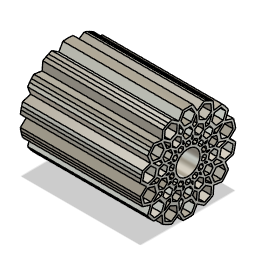
chevron + honeycomb v2 (Autodesk Fusion 360 archive; units mm, degrees)
design "honeycomb support"
Autodesk Fusion 360 part; units mm, degrees
sketch "Sketch1" plane through (0, 0, 0) normal (1, 0, 0) x (0, 0, -1)
  circle A0 centre (0, 0) radius 5
  circle A1 centre (0, 0) radius 20
  line L0 (0, 20.0404) -> (0, 18.9404) construction
  line L1 (0, 0) -> (0, 38.9808) construction
  line L2 (0, 13.1782) -> (0, 12.6782) construction
  line L3 (0, 8.1981) -> (0, 7.9981) construction
  line L4 (0, 5) -> (0, 5.5) construction
  line L5 (0, 8.0981) -> (0, 8.5981) construction
  line L6 (0, 12.9282) -> (0, 13.3) construction
  line L7 (0, 12.9282) -> (0, 13.4282) construction
  circle A2 centre (0, 0) radius 6
  line L8 (3.5471, 15.5409) -> (2.0387, 12.9282)
  line L9 (-2.0387, 12.9282) -> (-3.5471, 15.5409)
  line L10 (-3.8476, 16.8573) -> (-2.0968, 19.8898)
  line L11 (2.0968, 19.8898) -> (3.8476, 16.8573)
  line L12 (-2.6325, 11.5337) -> (-1.933, 12.7452)
  line L13 (1.933, 12.7452) -> (2.6325, 11.5337)
  line L14 (-1.7007, 7.4514) -> (-1.433, 7.9151)
  line L15 (1.433, 7.9151) -> (1.7007, 7.4514)
  line L16 (1.4613, 13.9282) -> (-1.4613, 13.9282)
  line L17 (-1.4613, 13.9282) -> (-2.9226, 16.4593)
  line L18 (-2.9226, 16.4593) -> (-1.4613, 18.9904)
  line L19 (-1.4613, 18.9904) -> (1.4613, 18.9904)
  line L20 (1.4613, 18.9904) -> (2.9226, 16.4593)
  line L21 (2.9226, 16.4593) -> (1.4613, 13.9282)
  line L22 (1.0191, 8.9981) -> (-1.0191, 8.9981)
  line L23 (-1.0191, 8.9981) -> (-2.0381, 10.7631)
  line L24 (-2.0381, 10.7631) -> (-1.0191, 12.5282)
  line L25 (-1.0191, 12.5282) -> (1.0191, 12.5282)
  line L26 (1.0191, 12.5282) -> (2.0381, 10.7631)
  line L27 (2.0381, 10.7631) -> (1.0191, 8.9981)
  line L28 (-0.6706, 5.9624) -> (-1.1536, 6.799)
  line L29 (-1.1536, 6.799) -> (-0.5768, 7.7981)
  line L30 (-0.5768, 7.7981) -> (0.5768, 7.7981)
  line L31 (0.5768, 7.7981) -> (1.1536, 6.799)
  line L32 (1.1536, 6.799) -> (0.6706, 5.9624)
  line L33 (1.5387, 8.0981) -> (1.4302, 7.9102)
  line L34 (1.5387, 8.0981) -> (1.7557, 8.0981) construction
  line L35 (-1.5387, 8.0981) -> (-1.433, 7.9151)
  line L36 (-1.5387, 8.0981) -> (-1.3274, 8.0981) construction
  line L37 (-2.0387, 12.9282) -> (-1.9268, 12.7345)
  line L38 (-2.0387, 12.9282) -> (-1.815, 12.9282) construction
  line L39 (2.0387, 12.9282) -> (1.933, 12.7452)
  line L40 (-7.4461, 10.7634) -> (-7.2613, 10.6374)
  line L41 (-7.4461, 10.7634) -> (-9.9388, 12.4628)
  line L42 (-10.7806, 13.5185) -> (-10.5103, 17.1262)
  line L43 (-10.5103, 17.1262) -> (-6.8367, 18.8953)
  line L44 (-6.8367, 18.8953) -> (-3.8476, 16.8573)
  line L45 (-3.7726, 12.5325) -> (-3.7883, 12.3217)
  line L46 (-3.7883, 12.3217) -> (-2.6325, 11.5337)
  line L47 (-2.1273, 7.9637) -> (-2.1435, 7.7473)
  line L48 (-3.5471, 15.5409) -> (-3.7726, 12.5325)
  line L49 (-2.1431, 7.753) -> (-1.7007, 7.4514)
  line L50 (-4.7653, 5.9755) -> (-4.7253, 6.5095)
  line L51 (-4.8999, 6.6285) -> (-4.7253, 6.5095)
  line L52 (-7.3761, 9.2493) -> (-7.2715, 10.6443)
  line L53 (-4.5176, 11.7297) -> (-2.8337, 10.5816)
  line L54 (-2.8337, 10.5816) -> (-2.986, 8.5491)
  line L55 (-2.986, 8.5491) -> (-4.8223, 7.6648)
  line L56 (-4.8223, 7.6648) -> (-6.5062, 8.8129)
  line L57 (-6.3539, 10.8454) -> (-4.5176, 11.7297)
  line L58 (-6.5062, 8.8129) -> (-6.3539, 10.8454)
  line L59 (-9.5562, 16.4757) -> (-6.923, 17.7438)
  line L60 (-6.923, 17.7438) -> (-4.5082, 16.0974)
  line L61 (-4.5082, 16.0974) -> (-4.7266, 13.1829)
  line L62 (-4.7266, 13.1829) -> (-7.3598, 11.9148)
  line L63 (-9.7746, 13.5612) -> (-9.5562, 16.4757)
  line L64 (-7.3598, 11.9148) -> (-9.7746, 13.5612)
  line L65 (-2.8638, 7.2761) -> (-1.9106, 6.6262)
  line L66 (-1.9106, 6.6262) -> (-1.9828, 5.6629)
  line L67 (-3.1911, 5.081) -> (-3.9893, 5.6252)
  line L68 (-3.9031, 6.7756) -> (-2.8638, 7.2761)
  line L69 (-3.9893, 5.6252) -> (-3.9031, 6.7756)
  line L70 (-11.3788, 6.4667) -> (-11.1576, 6.4334)
  line L71 (-11.3788, 6.4667) -> (-14.3619, 6.9163)
  line L72 (-15.5785, 7.5022) -> (-16.9002, 10.8699)
  line L73 (-16.9002, 10.8699) -> (-14.358, 14.0577)
  line L74 (-14.358, 14.0577) -> (-10.7806, 13.5185)
  line L75 (-8.8366, 9.6545) -> (-8.7594, 9.4578)
  line L76 (-8.7594, 9.4578) -> (-7.3761, 9.2493)
  line L77 (-5.372, 6.2521) -> (-5.2927, 6.0501)
  line L78 (-9.9388, 12.4628) -> (-8.8366, 9.6545)
  line L79 (-5.2948, 6.0553) -> (-4.7653, 5.9755)
  line L80 (-6.8861, 3.3162) -> (-7.0817, 3.8146)
  line L81 (-7.2907, 3.8461) -> (-7.0817, 3.8146)
  line L82 (-10.6587, 5.133) -> (-11.1698, 6.4352)
  line L83 (-9.1596, 8.6079) -> (-7.1442, 8.3042)
  line L84 (-7.1442, 8.3042) -> (-6.3996, 6.4069)
  line L85 (-6.3996, 6.4069) -> (-7.6704, 4.8135)
  line L86 (-7.6704, 4.8135) -> (-9.6857, 5.1172)
  line L87 (-10.4303, 7.0145) -> (-9.1596, 8.6079)
  line L88 (-9.6857, 5.1172) -> (-10.4303, 7.0145)
  line L89 (-15.7584, 10.6978) -> (-13.9362, 12.9828)
  line L90 (-13.9362, 12.9828) -> (-11.0462, 12.5472)
  line L91 (-11.0462, 12.5472) -> (-9.9784, 9.8266)
  line L92 (-9.9784, 9.8266) -> (-11.8006, 7.5416)
  line L93 (-14.6906, 7.9772) -> (-15.7584, 10.6978)
  line L94 (-11.8006, 7.5416) -> (-14.6906, 7.9772)
  line L95 (-5.7372, 5.313) -> (-4.5965, 5.141)
  line L96 (-4.5965, 5.141) -> (-4.2435, 4.2418)
  line L97 (-5.0797, 3.1932) -> (-6.035, 3.3372)
  line L98 (-6.4564, 4.4111) -> (-5.7372, 5.313)
  line L99 (-6.035, 3.3372) -> (-6.4564, 4.4111)
  line L100 (-13.0577, 0.8892) -> (-12.844, 0.9552)
  line L101 (-13.0577, 0.8892) -> (-15.9405, 0)
  line L102 (-17.2908, 0) -> (-19.9428, 2.4607)
  line L103 (-19.9428, 2.4607) -> (-19.0355, 6.4358)
  line L104 (-19.0355, 6.4358) -> (-15.5785, 7.5022)
  line L105 (-12.1504, 4.8644) -> (-11.9955, 4.7206)
  line L106 (-11.9955, 4.7206) -> (-10.6587, 5.133)
  line L107 (-7.5527, 3.3021) -> (-7.3936, 3.1545)
  line L108 (-14.3619, 6.9163) -> (-12.1504, 4.8644)
  line L109 (-7.3977, 3.1584) -> (-6.8861, 3.3162)
  line L110 (-7.643, 0) -> (-8.0355, 0.3642)
  line L111 (-8.2374, 0.3019) -> (-8.0355, 0.3642)
  line L112 (-11.8303, 0) -> (-12.8558, 0.9515)
  line L113 (-11.9873, 3.7813) -> (-10.0398, 4.382)
  line L114 (-10.0398, 4.382) -> (-8.5457, 2.9958)
  line L115 (-8.5457, 2.9958) -> (-8.9992, 1.0088)
  line L116 (-8.9992, 1.0088) -> (-10.9468, 0.408)
  line L117 (-12.4409, 1.7943) -> (-11.9873, 3.7813)
  line L118 (-10.9468, 0.408) -> (-12.4409, 1.7943)
  line L119 (-18.8394, 2.8011) -> (-18.1891, 5.6504)
  line L120 (-18.1891, 5.6504) -> (-15.3963, 6.5119)
  line L121 (-15.3963, 6.5119) -> (-13.2538, 4.524)
  line L122 (-13.2538, 4.524) -> (-13.9042, 1.6746)
  line L123 (-16.697, 0.8132) -> (-18.8394, 2.8011)
  line L124 (-13.9042, 1.6746) -> (-16.697, 0.8132)
  line L125 (-7.4742, 2.2976) -> (-6.3719, 2.6376)
  line L126 (-6.3719, 2.6376) -> (-5.6637, 1.9805)
  line L127 (-5.9621, 0.673) -> (-6.8853, 0.3883)
  line L128 (-7.7309, 1.1729) -> (-7.4742, 2.2976)
  line L129 (-6.8853, 0.3883) -> (-7.7309, 1.1729)
  line L130 (-12.1504, -4.8644) -> (-11.9864, -4.7122)
  line L131 (-12.1504, -4.8644) -> (-14.3619, -6.9163)
  line L132 (-15.5785, -7.5022) -> (-19.0355, -6.4358)
  line L133 (-19.0355, -6.4358) -> (-19.9428, -2.4607)
  line L134 (-19.9428, -2.4607) -> (-17.2908, 0)
  line L135 (-13.0577, -0.8892) -> (-12.8558, -0.9515)
  line L136 (-12.8558, -0.9515) -> (-11.8303, 0)
  line L137 (-8.2374, -0.3019) -> (-8.0301, -0.3659)
  line L138 (-15.9405, 0) -> (-13.0577, -0.8892)
  line L139 (-8.0355, -0.3642) -> (-7.643, 0)
  line L140 (-6.8861, -3.3162) -> (-7.3977, -3.1584)
  line L141 (-7.5527, -3.3021) -> (-7.3977, -3.1584)
  line L142 (-10.6587, -5.133) -> (-11.9955, -4.7206)
  line L143 (-12.4409, -1.7943) -> (-10.9468, -0.408)
  line L144 (-10.9468, -0.408) -> (-8.9992, -1.0088)
  line L145 (-8.9992, -1.0088) -> (-8.5457, -2.9958)
  line L146 (-8.5457, -2.9958) -> (-10.0398, -4.382)
  line L147 (-11.9873, -3.7813) -> (-12.4409, -1.7943)
  line L148 (-10.0398, -4.382) -> (-11.9873, -3.7813)
  line L149 (-18.1891, -5.6504) -> (-18.8394, -2.8011)
  line L150 (-18.8394, -2.8011) -> (-16.697, -0.8132)
  line L151 (-16.697, -0.8132) -> (-13.9042, -1.6746)
  line L152 (-13.9042, -1.6746) -> (-13.2538, -4.524)
  line L153 (-15.3963, -6.5119) -> (-18.1891, -5.6504)
  line L154 (-13.2538, -4.524) -> (-15.3963, -6.5119)
  line L155 (-7.7309, -1.1729) -> (-6.8853, -0.3883)
  line L156 (-6.8853, -0.3883) -> (-5.9621, -0.673)
  line L157 (-5.6637, -1.9805) -> (-6.3719, -2.6376)
  line L158 (-7.4742, -2.2976) -> (-7.7309, -1.1729)
  line L159 (-6.3719, -2.6376) -> (-7.4742, -2.2976)
  line L160 (-8.8366, -9.6545) -> (-8.7549, -9.4463)
  line L161 (-8.8366, -9.6545) -> (-9.9388, -12.4628)
  line L162 (-10.7806, -13.5185) -> (-14.358, -14.0577)
  line L163 (-14.358, -14.0577) -> (-16.9002, -10.8699)
  line L164 (-16.9002, -10.8699) -> (-15.5785, -7.5022)
  line L165 (-11.3788, -6.4667) -> (-11.1698, -6.4352)
  line L166 (-11.1698, -6.4352) -> (-10.6587, -5.133)
  line L167 (-7.2907, -3.8461) -> (-7.0761, -3.8137)
  line L168 (-14.3619, -6.9163) -> (-11.3788, -6.4667)
  line L169 (-7.0817, -3.8146) -> (-6.8861, -3.3162)
  line L170 (-4.7653, -5.9755) -> (-5.2948, -6.0553)
  line L171 (-5.372, -6.2521) -> (-5.2948, -6.0553)
  line L172 (-7.3761, -9.2493) -> (-8.7594, -9.4578)
  line L173 (-10.4303, -7.0145) -> (-9.6857, -5.1172)
  line L174 (-9.6857, -5.1172) -> (-7.6704, -4.8135)
  line L175 (-7.6704, -4.8135) -> (-6.3996, -6.4069)
  line L176 (-6.3996, -6.4069) -> (-7.1442, -8.3042)
  line L177 (-9.1596, -8.6079) -> (-10.4303, -7.0145)
  line L178 (-7.1442, -8.3042) -> (-9.1596, -8.6079)
  line L179 (-13.9362, -12.9828) -> (-15.7584, -10.6978)
  line L180 (-15.7584, -10.6978) -> (-14.6906, -7.9772)
  line L181 (-14.6906, -7.9772) -> (-11.8006, -7.5416)
  line L182 (-11.8006, -7.5416) -> (-9.9784, -9.8266)
  line L183 (-11.0462, -12.5472) -> (-13.9362, -12.9828)
  line L184 (-9.9784, -9.8266) -> (-11.0462, -12.5472)
  line L185 (-6.4564, -4.4111) -> (-6.035, -3.3372)
  line L186 (-6.035, -3.3372) -> (-5.0797, -3.1932)
  line L187 (-4.2435, -4.2418) -> (-4.5965, -5.141)
  line L188 (-5.7372, -5.313) -> (-6.4564, -4.4111)
  line L189 (-4.5965, -5.141) -> (-5.7372, -5.313)
  line L190 (-3.7726, -12.5325) -> (-3.7893, -12.3094)
  line L191 (-3.7726, -12.5325) -> (-3.5471, -15.5409)
  line L192 (-3.8476, -16.8573) -> (-6.8367, -18.8953)
  line L193 (-6.8367, -18.8953) -> (-10.5103, -17.1262)
  line L194 (-10.5103, -17.1262) -> (-10.7806, -13.5185)
  line L195 (-7.4461, -10.7634) -> (-7.2715, -10.6443)
  line L196 (-7.2715, -10.6443) -> (-7.3761, -9.2493)
  line L197 (-4.8999, -6.6285) -> (-4.7206, -6.5063)
  line L198 (-9.9388, -12.4628) -> (-7.4461, -10.7634)
  line L199 (-4.7253, -6.5095) -> (-4.7653, -5.9755)
  line L200 (-1.7007, -7.4514) -> (-2.1431, -7.753)
  line L201 (-2.1273, -7.9637) -> (-2.1431, -7.753)
  line L202 (-2.6325, -11.5337) -> (-3.7883, -12.3217)
  line L203 (-6.3539, -10.8454) -> (-6.5062, -8.8129)
  line L204 (-6.5062, -8.8129) -> (-4.8223, -7.6648)
  line L205 (-4.8223, -7.6648) -> (-2.986, -8.5491)
  line L206 (-2.986, -8.5491) -> (-2.8337, -10.5816)
  line L207 (-4.5176, -11.7297) -> (-6.3539, -10.8454)
  line L208 (-2.8337, -10.5816) -> (-4.5176, -11.7297)
  line L209 (-6.923, -17.7438) -> (-9.5562, -16.4757)
  line L210 (-9.5562, -16.4757) -> (-9.7746, -13.5612)
  line L211 (-9.7746, -13.5612) -> (-7.3598, -11.9148)
  line L212 (-7.3598, -11.9148) -> (-4.7266, -13.1829)
  line L213 (-4.5082, -16.0974) -> (-6.923, -17.7438)
  line L214 (-4.7266, -13.1829) -> (-4.5082, -16.0974)
  line L215 (-3.9031, -6.7756) -> (-3.9893, -5.6252)
  line L216 (-3.9893, -5.6252) -> (-3.1911, -5.081)
  line L217 (-1.9828, -5.6629) -> (-1.9106, -6.6262)
  line L218 (-2.8638, -7.2761) -> (-3.9031, -6.7756)
  line L219 (-1.9106, -6.6262) -> (-2.8638, -7.2761)
  line L220 (2.0387, -12.9282) -> (1.9268, -12.7345)
  line L221 (2.0387, -12.9282) -> (3.5471, -15.5409)
  line L222 (3.8476, -16.8573) -> (2.0387, -19.9904)
  line L223 (2.0387, -19.9904) -> (-2.0387, -19.9904)
  line L224 (-2.0387, -19.9904) -> (-3.8476, -16.8573)
  line L225 (-2.0387, -12.9282) -> (-1.933, -12.7452)
  line L226 (-1.933, -12.7452) -> (-2.6325, -11.5337)
  line L227 (-1.5387, -8.0981) -> (-1.4302, -7.9102)
  line L228 (-3.5471, -15.5409) -> (-2.0387, -12.9282)
  line L229 (-1.433, -7.9151) -> (-1.7007, -7.4514)
  line L230 (1.7007, -7.4514) -> (1.433, -7.9151)
  line L231 (1.5387, -8.0981) -> (1.433, -7.9151)
  line L232 (2.6325, -11.5337) -> (1.933, -12.7452)
  line L233 (-1.0191, -12.5282) -> (-2.0381, -10.7631)
  line L234 (-2.0381, -10.7631) -> (-1.0191, -8.9981)
  line L235 (-1.0191, -8.9981) -> (1.0191, -8.9981)
  line L236 (1.0191, -8.9981) -> (2.0381, -10.7631)
  line L237 (1.0191, -12.5282) -> (-1.0191, -12.5282)
  line L238 (2.0381, -10.7631) -> (1.0191, -12.5282)
  line L239 (1.4613, -18.9904) -> (-1.4613, -18.9904)
  line L240 (-1.4613, -18.9904) -> (-2.9226, -16.4593)
  line L241 (-2.9226, -16.4593) -> (-1.4613, -13.9282)
  line L242 (-1.4613, -13.9282) -> (1.4613, -13.9282)
  line L243 (2.9226, -16.4593) -> (1.4613, -18.9904)
  line L244 (1.4613, -13.9282) -> (2.9226, -16.4593)
  line L245 (-0.5768, -7.7981) -> (-1.1536, -6.799)
  line L246 (-1.1536, -6.799) -> (-0.6706, -5.9624)
  line L247 (0.6706, -5.9624) -> (1.1536, -6.799)
  line L248 (0.5768, -7.7981) -> (-0.5768, -7.7981)
  line L249 (1.1536, -6.799) -> (0.5768, -7.7981)
  line L250 (7.4461, -10.7634) -> (7.2613, -10.6374)
  line L251 (7.4461, -10.7634) -> (9.9388, -12.4628)
  line L252 (10.7806, -13.5185) -> (10.5103, -17.1262)
  line L253 (10.5103, -17.1262) -> (6.8367, -18.8953)
  line L254 (6.8367, -18.8953) -> (3.8476, -16.8573)
  line L255 (3.7726, -12.5325) -> (3.7883, -12.3217)
  line L256 (3.7883, -12.3217) -> (2.6325, -11.5337)
  line L257 (2.1273, -7.9637) -> (2.1435, -7.7473)
  line L258 (3.5471, -15.5409) -> (3.7726, -12.5325)
  line L259 (2.1431, -7.753) -> (1.7007, -7.4514)
  line L260 (4.7653, -5.9755) -> (4.7253, -6.5095)
  line L261 (4.8999, -6.6285) -> (4.7253, -6.5095)
  line L262 (7.3761, -9.2493) -> (7.2715, -10.6443)
  line L263 (4.5176, -11.7297) -> (2.8337, -10.5816)
  line L264 (2.8337, -10.5816) -> (2.986, -8.5491)
  line L265 (2.986, -8.5491) -> (4.8223, -7.6648)
  line L266 (4.8223, -7.6648) -> (6.5062, -8.8129)
  line L267 (6.3539, -10.8454) -> (4.5176, -11.7297)
  line L268 (6.5062, -8.8129) -> (6.3539, -10.8454)
  line L269 (9.5562, -16.4757) -> (6.923, -17.7438)
  line L270 (6.923, -17.7438) -> (4.5082, -16.0974)
  line L271 (4.5082, -16.0974) -> (4.7266, -13.1829)
  line L272 (4.7266, -13.1829) -> (7.3598, -11.9148)
  line L273 (9.7746, -13.5612) -> (9.5562, -16.4757)
  line L274 (7.3598, -11.9148) -> (9.7746, -13.5612)
  line L275 (2.8638, -7.2761) -> (1.9106, -6.6262)
  line L276 (1.9106, -6.6262) -> (1.9828, -5.6629)
  line L277 (3.1911, -5.081) -> (3.9893, -5.6252)
  line L278 (3.9031, -6.7756) -> (2.8638, -7.2761)
  line L279 (3.9893, -5.6252) -> (3.9031, -6.7756)
  line L280 (11.3788, -6.4667) -> (11.1576, -6.4334)
  line L281 (11.3788, -6.4667) -> (14.3619, -6.9163)
  line L282 (15.5785, -7.5022) -> (16.9002, -10.8699)
  line L283 (16.9002, -10.8699) -> (14.358, -14.0577)
  line L284 (14.358, -14.0577) -> (10.7806, -13.5185)
  line L285 (8.8366, -9.6545) -> (8.7594, -9.4578)
  line L286 (8.7594, -9.4578) -> (7.3761, -9.2493)
  line L287 (5.372, -6.2521) -> (5.2927, -6.0501)
  line L288 (9.9388, -12.4628) -> (8.8366, -9.6545)
  line L289 (5.2948, -6.0553) -> (4.7653, -5.9755)
  line L290 (6.8861, -3.3162) -> (7.0817, -3.8146)
  line L291 (7.2907, -3.8461) -> (7.0817, -3.8146)
  line L292 (10.6587, -5.133) -> (11.1698, -6.4352)
  line L293 (9.1596, -8.6079) -> (7.1442, -8.3042)
  line L294 (7.1442, -8.3042) -> (6.3996, -6.4069)
  line L295 (6.3996, -6.4069) -> (7.6704, -4.8135)
  line L296 (7.6704, -4.8135) -> (9.6857, -5.1172)
  line L297 (10.4303, -7.0145) -> (9.1596, -8.6079)
  line L298 (9.6857, -5.1172) -> (10.4303, -7.0145)
  line L299 (15.7584, -10.6978) -> (13.9362, -12.9828)
  line L300 (13.9362, -12.9828) -> (11.0462, -12.5472)
  line L301 (11.0462, -12.5472) -> (9.9784, -9.8266)
  line L302 (9.9784, -9.8266) -> (11.8006, -7.5416)
  line L303 (14.6906, -7.9772) -> (15.7584, -10.6978)
  line L304 (11.8006, -7.5416) -> (14.6906, -7.9772)
  line L305 (5.7372, -5.313) -> (4.5965, -5.141)
  line L306 (4.5965, -5.141) -> (4.2435, -4.2418)
  line L307 (5.0797, -3.1932) -> (6.035, -3.3372)
  line L308 (6.4564, -4.4111) -> (5.7372, -5.313)
  line L309 (6.035, -3.3372) -> (6.4564, -4.4111)
  line L310 (13.0577, -0.8892) -> (12.844, -0.9552)
  line L311 (13.0577, -0.8892) -> (15.9405, 0)
  line L312 (17.2908, 0) -> (19.9428, -2.4607)
  line L313 (19.9428, -2.4607) -> (19.0355, -6.4358)
  line L314 (19.0355, -6.4358) -> (15.5785, -7.5022)
  line L315 (12.1504, -4.8644) -> (11.9955, -4.7206)
  line L316 (11.9955, -4.7206) -> (10.6587, -5.133)
  line L317 (7.5527, -3.3021) -> (7.3936, -3.1545)
  line L318 (14.3619, -6.9163) -> (12.1504, -4.8644)
  line L319 (7.3977, -3.1584) -> (6.8861, -3.3162)
  line L320 (7.643, 0) -> (8.0355, -0.3642)
  line L321 (8.2374, -0.3019) -> (8.0355, -0.3642)
  line L322 (11.8303, 0) -> (12.8558, -0.9515)
  line L323 (11.9873, -3.7813) -> (10.0398, -4.382)
  line L324 (10.0398, -4.382) -> (8.5457, -2.9958)
  line L325 (8.5457, -2.9958) -> (8.9992, -1.0088)
  line L326 (8.9992, -1.0088) -> (10.9468, -0.408)
  line L327 (12.4409, -1.7943) -> (11.9873, -3.7813)
  line L328 (10.9468, -0.408) -> (12.4409, -1.7943)
  line L329 (18.8394, -2.8011) -> (18.1891, -5.6504)
  line L330 (18.1891, -5.6504) -> (15.3963, -6.5119)
  line L331 (15.3963, -6.5119) -> (13.2538, -4.524)
  line L332 (13.2538, -4.524) -> (13.9042, -1.6746)
  line L333 (16.697, -0.8132) -> (18.8394, -2.8011)
  line L334 (13.9042, -1.6746) -> (16.697, -0.8132)
  line L335 (7.4742, -2.2976) -> (6.3719, -2.6376)
  line L336 (6.3719, -2.6376) -> (5.6637, -1.9805)
  line L337 (5.9621, -0.673) -> (6.8853, -0.3883)
  line L338 (7.7309, -1.1729) -> (7.4742, -2.2976)
  line L339 (6.8853, -0.3883) -> (7.7309, -1.1729)
  line L340 (12.1504, 4.8644) -> (11.9864, 4.7122)
  line L341 (12.1504, 4.8644) -> (14.3619, 6.9163)
  line L342 (15.5785, 7.5022) -> (19.0355, 6.4358)
  line L343 (19.0355, 6.4358) -> (19.9428, 2.4607)
  line L344 (19.9428, 2.4607) -> (17.2908, 0)
  line L345 (13.0577, 0.8892) -> (12.8558, 0.9515)
  line L346 (12.8558, 0.9515) -> (11.8303, 0)
  line L347 (8.2374, 0.3019) -> (8.0301, 0.3659)
  line L348 (15.9405, 0) -> (13.0577, 0.8892)
  line L349 (8.0355, 0.3642) -> (7.643, 0)
  line L350 (6.8861, 3.3162) -> (7.3977, 3.1584)
  line L351 (7.5527, 3.3021) -> (7.3977, 3.1584)
  line L352 (10.6587, 5.133) -> (11.9955, 4.7206)
  line L353 (12.4409, 1.7943) -> (10.9468, 0.408)
  line L354 (10.9468, 0.408) -> (8.9992, 1.0088)
  line L355 (8.9992, 1.0088) -> (8.5457, 2.9958)
  line L356 (8.5457, 2.9958) -> (10.0398, 4.382)
  line L357 (11.9873, 3.7813) -> (12.4409, 1.7943)
  line L358 (10.0398, 4.382) -> (11.9873, 3.7813)
  line L359 (18.1891, 5.6504) -> (18.8394, 2.8011)
  line L360 (18.8394, 2.8011) -> (16.697, 0.8132)
  line L361 (16.697, 0.8132) -> (13.9042, 1.6746)
  line L362 (13.9042, 1.6746) -> (13.2538, 4.524)
  line L363 (15.3963, 6.5119) -> (18.1891, 5.6504)
  line L364 (13.2538, 4.524) -> (15.3963, 6.5119)
  line L365 (7.7309, 1.1729) -> (6.8853, 0.3883)
  line L366 (6.8853, 0.3883) -> (5.9621, 0.673)
  line L367 (5.6637, 1.9805) -> (6.3719, 2.6376)
  line L368 (7.4742, 2.2976) -> (7.7309, 1.1729)
  line L369 (6.3719, 2.6376) -> (7.4742, 2.2976)
  line L370 (8.8366, 9.6545) -> (8.7549, 9.4463)
  line L371 (8.8366, 9.6545) -> (9.9388, 12.4628)
  line L372 (10.7806, 13.5185) -> (14.358, 14.0577)
  line L373 (14.358, 14.0577) -> (16.9002, 10.8699)
  line L374 (16.9002, 10.8699) -> (15.5785, 7.5022)
  line L375 (11.3788, 6.4667) -> (11.1698, 6.4352)
  line L376 (11.1698, 6.4352) -> (10.6587, 5.133)
  line L377 (7.2907, 3.8461) -> (7.0761, 3.8137)
  line L378 (14.3619, 6.9163) -> (11.3788, 6.4667)
  line L379 (7.0817, 3.8146) -> (6.8861, 3.3162)
  line L380 (4.7653, 5.9755) -> (5.2948, 6.0553)
  line L381 (5.372, 6.2521) -> (5.2948, 6.0553)
  line L382 (7.3761, 9.2493) -> (8.7594, 9.4578)
  line L383 (10.4303, 7.0145) -> (9.6857, 5.1172)
  line L384 (9.6857, 5.1172) -> (7.6704, 4.8135)
  line L385 (7.6704, 4.8135) -> (6.3996, 6.4069)
  line L386 (6.3996, 6.4069) -> (7.1442, 8.3042)
  line L387 (9.1596, 8.6079) -> (10.4303, 7.0145)
  line L388 (7.1442, 8.3042) -> (9.1596, 8.6079)
  line L389 (13.9362, 12.9828) -> (15.7584, 10.6978)
  line L390 (15.7584, 10.6978) -> (14.6906, 7.9772)
  line L391 (14.6906, 7.9772) -> (11.8006, 7.5416)
  line L392 (11.8006, 7.5416) -> (9.9784, 9.8266)
  line L393 (11.0462, 12.5472) -> (13.9362, 12.9828)
  line L394 (9.9784, 9.8266) -> (11.0462, 12.5472)
  line L395 (6.4564, 4.4111) -> (6.035, 3.3372)
  line L396 (6.035, 3.3372) -> (5.0797, 3.1932)
  line L397 (4.2435, 4.2418) -> (4.5965, 5.141)
  line L398 (5.7372, 5.313) -> (6.4564, 4.4111)
  line L399 (4.5965, 5.141) -> (5.7372, 5.313)
  line L400 (3.7726, 12.5325) -> (3.7893, 12.3094)
  line L401 (3.7726, 12.5325) -> (3.5471, 15.5409)
  line L402 (3.8476, 16.8573) -> (6.8367, 18.8953)
  line L403 (6.8367, 18.8953) -> (10.5103, 17.1262)
  line L404 (10.5103, 17.1262) -> (10.7806, 13.5185)
  line L405 (7.4461, 10.7634) -> (7.2715, 10.6443)
  line L406 (7.2715, 10.6443) -> (7.3761, 9.2493)
  line L407 (4.8999, 6.6285) -> (4.7206, 6.5063)
  line L408 (9.9388, 12.4628) -> (7.4461, 10.7634)
  line L409 (1.7007, 7.4514) -> (2.1431, 7.753)
  line L410 (2.1273, 7.9637) -> (2.1431, 7.753)
  line L411 (2.6325, 11.5337) -> (3.7883, 12.3217)
  line L412 (6.3539, 10.8454) -> (6.5062, 8.8129)
  line L413 (6.5062, 8.8129) -> (4.8223, 7.6648)
  line L414 (4.8223, 7.6648) -> (2.986, 8.5491)
  line L415 (2.986, 8.5491) -> (2.8337, 10.5816)
  line L416 (4.5176, 11.7297) -> (6.3539, 10.8454)
  line L417 (2.8337, 10.5816) -> (4.5176, 11.7297)
  line L418 (6.923, 17.7438) -> (9.5562, 16.4757)
  line L419 (9.5562, 16.4757) -> (9.7746, 13.5612)
  line L420 (9.7746, 13.5612) -> (7.3598, 11.9148)
  line L421 (7.3598, 11.9148) -> (4.7266, 13.1829)
  line L422 (4.5082, 16.0974) -> (6.923, 17.7438)
  line L423 (4.7266, 13.1829) -> (4.5082, 16.0974)
  line L424 (3.9031, 6.7756) -> (3.9893, 5.6252)
  line L425 (3.9893, 5.6252) -> (3.1911, 5.081)
  line L426 (2.8638, 7.2761) -> (3.9031, 6.7756)
  line L427 (1.9106, 6.6262) -> (2.8638, 7.2761)
  line L428 (7.2907, -3.8461) -> (8.3035, -3.9987)
  line L429 (8.3035, -3.9987) -> (7.5527, -3.3021)
  line L430 (5.7462, -7.2055) -> (5.372, -6.2521)
  line L431 (4.8999, -6.6285) -> (5.7462, -7.2055)
  line L432 (-5.7462, -7.2055) -> (-4.8999, -6.6285)
  line L433 (-5.372, -6.2521) -> (-5.7462, -7.2055)
  line L434 (-7.5527, -3.3021) -> (-8.3035, -3.9987)
  line L435 (-8.3035, -3.9987) -> (-7.2907, -3.8461)
  line L436 (-9.2161, 0) -> (-8.2374, -0.3019)
  line L437 (-8.2374, 0.3019) -> (-9.2161, 0)
  line L438 (-7.0908, 0.5123) -> (-6.9832, 0.4791)
  line L439 (-2.1273, -7.9637) -> (-2.0508, -8.9851)
  line L440 (-2.0508, -8.9851) -> (-1.5387, -8.0981)
  line L441 (2.0508, -8.9851) -> (2.1273, -7.9637)
  line L442 (1.5387, -8.0981) -> (2.0508, -8.9851)
  line L443 (7.5527, 3.3021) -> (8.3035, 3.9987)
  line L444 (8.3035, 3.9987) -> (7.2907, 3.8461)
  line L445 (8.2374, -0.3019) -> (9.2161, 0)
  line L446 (9.2161, 0) -> (8.2374, 0.3019)
  line L447 (5.372, 6.2521) -> (5.7462, 7.2055)
  line L448 (5.7462, 7.2055) -> (4.8999, 6.6285)
  line L449 (4.7253, 6.5095) -> (4.7653, 5.9755)
  line L450 (3.8779, 5.5) -> (3.9043, 5.5672)
  line L451 (-1.5387, 8.0981) -> (-2.0508, 8.9851)
  line L452 (-2.0508, 8.9851) -> (-2.1273, 7.9637)
  line L453 (2.0508, 8.9851) -> (1.5387, 8.0981)
  line L454 (2.1273, 7.9637) -> (2.0508, 8.9851)
  line L455 (-5.7462, 7.2055) -> (-5.372, 6.2521)
  line L456 (-4.8999, 6.6285) -> (-5.7462, 7.2055)
  line L457 (-7.2907, 3.8461) -> (-8.3035, 3.9987)
  line L458 (-8.3035, 3.9987) -> (-7.5527, 3.3021)
  line L459 (1.9969, 5.4759) -> (1.995, 5.5)
  line L460 (1.9828, 5.6629) -> (1.9106, 6.6262)
  line L461 (-0.75, 5.5) -> (0, 5.5) construction
  line L462 (1.3274, 5.5) -> (11.4891, 5.5) construction
  dimension "d1" = 10
  dimension "d2" = 40
  dimension "d52" = 0.5
  dimension "d53" = 0.5
  dimension "d54" = 0.5
  dimension "d58" = 12
  dimension "d72" = 120
  dimension "d73" = 60
  dimension "d74" = 60
  constraint coincident A0.centre A1.centre
  constraint horizontal L461
  constraint midpoint L0 L1
  constraint coincident L1 L2.start
  constraint coincident L1 L2.end
  constraint coincident L1 L3.start
  constraint coincident L1 L3.end
  constraint coincident L1 L4.start
  constraint coincident A0 L4.start
  constraint midpoint L2 L6.start
  constraint coincident L1 L6.end
  constraint parallel L6 L7
  constraint concentric A0 A2
  constraint horizontal L34
  constraint horizontal L36
  constraint parallel L35 L451
  constraint horizontal L38
  constraint parallel L9 L37
  constraint parallel L8 L39
  constraint coincident L37 L12.end
  constraint coincident L33 L15.start
  constraint coincident A1 L11.start
  constraint coincident A1 L10.end
  constraint coincident L129 L438.end
  constraint coincident L425 L450.end
  constraint coincident L450.start L461
  constraint coincident A2 L66.end
  constraint coincident A2 L67.start
  constraint coincident A2 L96.end
  constraint coincident A2 L97.start
  constraint coincident A2 L127.start
  constraint coincident A2 L126.end
  constraint coincident A2 L156.end
  constraint coincident A2 L157.start
  constraint coincident A2 L186.end
  constraint coincident A2 L187.start
  constraint coincident A2 L216.end
  constraint coincident A2 L217.start
  constraint coincident A2 L246.end
  constraint coincident A2 L247.start
  constraint coincident A2 L276.end
  constraint coincident A2 L277.start
  constraint coincident A2 L306.end
  constraint coincident A2 L307.start
  constraint coincident A2 L336.end
  constraint coincident A2 L337.start
  constraint coincident A2 L366.end
  constraint coincident A2 L367.start
  constraint coincident A2 L396.end
  constraint coincident A2 L397.start
  constraint coincident A2 L425.end
  constraint coincident L459.end L461
  constraint coincident A2 L460.start
  constraint collinear L459 L460
  constraint coincident L462.start L461
  constraint collinear L461 L462
  constraint coincident A2 L32.end
  constraint coincident A2 L28.start
  measures "d1" diameter of A0
  measures "d2" diameter of A1
  measures "d52" distance of L4.start L4.end
  measures "d53" distance of L5.start L5.end
  measures "d54" distance of L6.start L7.end
  measures "d58" diameter of A2
  measures "d72" angle of L33 L34
  measures "d73" angle of L35 L36
  measures "d74" angle of L37 L38
extrude "Extrude1" add sketch "Sketch1" against normal blind 50 contours A1 L10 L11 L42 L43 L44 L72 L73 L74 L102 L103 L104 L132 L133 L134 L162 L163 L164 L192 L193 L194 L222 L223 L224 L252 L253 L254 L282 L283 L284 L312 L313 L314 L342 L343 L344 L372 L373 L374 L402 L403 L404
extrude "Extrude2" add sketch "Sketch1" against normal blind 50 contours A2

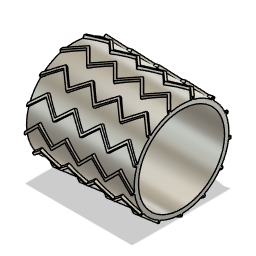
design "chevron tread"
Autodesk Fusion 360 part; units mm, degrees
sketch "Sketch1" plane through (0, 0, 0) normal (0, 1, 0) x (1, 0, 0)
  line L0 (-50, 22) -> (0, 22)
  line L1 (0, 22) -> (0, 20)
  line L2 (0, 20) -> (-50, 20)
  line L3 (-50, 20) -> (-50, 22)
  line L4 (0, 0) -> (0, 6) construction
  dimension "d1" = 50
  dimension "d2" = 2
  dimension "d3" = 20
  constraint horizontal L0
  constraint vertical L1
  constraint horizontal L2
  constraint vertical L3
  constraint coincident L4.start origin
  constraint vertical L4
  constraint collinear L1 L4
  measures "d1" distance of L1.end L2.end
  measures "d2" distance of L0.end L1.end
  measures "d3" distance of L4.start L1.end
revolve "Revolve1" add sketch "Sketch1" angle 360 about axis through (1.75, 0, 0) along (1, 0, 0)
sketch "Sketch3" plane through (0, 0, 0) normal (0, 0, 1) x (1, 0, 0)
  line L0 (0, 0) -> (0, -3.125) construction
  line L1 (0, -3.125) -> (-6.2497, 3.1247)
  line L2 (0, -3.125) -> (8.8384, -3.125) construction
  line L3 (-6.2497, 3.1247) -> (-12.4994, -3.125)
  line L4 (-12.4994, -3.125) -> (-18.749, 3.1247)
  line L5 (-18.749, 3.1247) -> (-24.9987, -3.125)
  line L6 (-24.9987, -3.125) -> (-31.2484, 3.1247)
  line L7 (-31.2484, 3.1247) -> (-37.4981, -3.125)
  line L8 (-37.4981, -3.125) -> (-43.7478, 3.1247)
  line L9 (-43.7478, 3.1247) -> (-49.9974, -3.125)
  line L10 (0.3536, -2.7714) -> (-6.2497, 3.8318)
  line L11 (-6.2497, 3.8318) -> (-12.4994, -2.4179)
  line L12 (-12.4994, -2.4179) -> (-18.749, 3.8318)
  line L13 (-18.749, 3.8318) -> (-24.9987, -2.4179)
  line L14 (-24.9987, -2.4179) -> (-31.2484, 3.8318)
  line L15 (-31.2484, 3.8318) -> (-37.4981, -2.4179)
  line L16 (-37.4981, -2.4179) -> (-43.7478, 3.8318)
  line L17 (-43.7478, 3.8318) -> (-50.6314, -3.0518)
  line L18 (-0.3536, -3.4786) -> (-6.2497, 2.4176)
  line L19 (-6.2497, 2.4176) -> (-12.4994, -3.8321)
  line L20 (-12.4994, -3.8321) -> (-18.749, 2.4176)
  line L21 (-18.749, 2.4176) -> (-24.9987, -3.8321)
  line L22 (-24.9987, -3.8321) -> (-31.2484, 2.4176)
  line L23 (-31.2484, 2.4176) -> (-37.4981, -3.8321)
  line L24 (-37.4981, -3.8321) -> (-43.7478, 2.4176)
  line L25 (-43.7478, 2.4176) -> (-49.9243, -3.7589)
  line L26 (-0.3536, -3.4786) -> (0.3536, -2.7714)
  line L27 (-49.9243, -3.7589) -> (-50.6314, -3.0518)
  dimension "d13" = 3.125
  dimension "d14" = 135
  dimension "d15" = 8.8384
  dimension "d16" = 8.8384
  dimension "d17" = 90
  dimension "d18" = 8.8384
  dimension "d19" = 8.8384
  dimension "d20" = 8.8384
  dimension "d21" = 8.8384
  dimension "d22" = 8.8384
  dimension "d23" = 8.8384
  dimension "d24" = 90
  dimension "d25" = 90
  dimension "d26" = 90
  dimension "d27" = 0.5
  dimension "d28" = -0.5
  constraint coincident L0.start origin
  constraint vertical L0
  constraint horizontal L2
  constraint parallel L4 L6
  constraint perpendicular L7 L8
  constraint coincident L3.end L4.start
  constraint perpendicular L10 L26
  constraint perpendicular L17 L27
  constraint perpendicular L3 L4
  measures "d13" distance of L0.start L0.end
  measures "d14" angle of L1 L2
  measures "d15" distance of L0.end L1.end
  measures "d16" distance of L1.end L3.end
  measures "d17" angle of L1 L3
  measures "d18" distance of L3.end L4.end
  measures "d19" distance of L4.end L5.end
  measures "d20" distance of L5.end L6.end
  measures "d21" distance of L6.end L7.end
  measures "d22" distance of L7.end L8.end
  measures "d23" distance of L8.end L9.end
  measures "d24" angle of L4 L5
  measures "d25" angle of L6 L7
  measures "d26" angle of L8 L9
extrude "Extrude1" add sketch "Sketch3" along normal blind 23
pattern_circular "C-Pattern1" count 13 over 360 about axis through (1.75, 0, 0) along (1, 0, 0) of "Extrude1"
sketch "Sketch4" plane through (0, 0, 0) normal (1, 0, 0) x (0, 0, -1)
  circle A0 centre (0, 0) radius 20
  circle A1 centre (0, 0) radius 25
  dimension "d33" = 40
  dimension "d38" = 50
  constraint coincident A0.centre A1.centre
  constraint concentric A0 A1
  measures "d33" diameter of A0
  measures "d38" diameter of A1
extrude "Extrude2" cut sketch "Sketch4" against normal blind 55 contours A0
extrude "Extrude3" cut sketch "Sketch4" along normal blind 5
extrude "Extrude4" cut sketch "Sketch4" along normal blind 5 contours A0
sketch "Sketch5" plane through (-50, 0, 0) normal (-1, 0, 0) x (0, 0, 1)
  line L0 (-16.4652, -11.3532) -> (-17.9723, -12.6884)
  arc A0 (18.2369, -12.305) -> (21.6895, -3.6832) centre (0, 0) ccw
  line L1 (16.4541, -11.3693) -> (18.2369, -12.305)
  arc A1 (16.4541, -11.3693) -> (19.6579, -3.6832) centre (0, 0) ccw
  circle A2 centre (0, 0) radius 25
  line L2 (21.6895, -3.6832) -> (19.6579, -3.6832)
  arc A3 (-17.9723, -12.6884) -> (-11.1351, -18.9739) centre (0, 0) ccw
  line L3 (-11.1351, -18.9739) -> (-10.4147, -17.0744)
  arc A4 (-16.4652, -11.3532) -> (-10.4147, -17.0744) centre (0, 0) ccw
  dimension "d41" = 50
  constraint coincident A0.centre A1.centre
  measures "d41" diameter of A2
extrude "Extrude5" cut sketch "Sketch5" along normal blind 9
equation "d16 = d15"
equation "d18 = d15"
equation "d19 = d15"
equation "d20 = d15"
equation "d21 = d15"
equation "d22 = d15"
equation "d23 = d15"
equation "d24 = d17"
equation "d25 = d17"
equation "d26 = d17"
